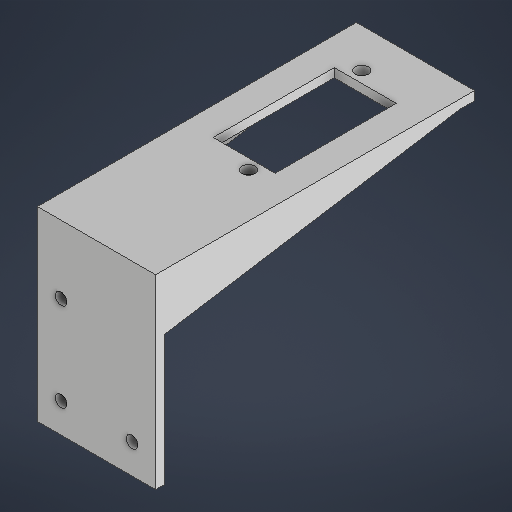
# Autodesk Inventor part: pan_base_holder_first_v1
Saved by Autodesk Inventor 2026 (Build 300175000, 175)
## iProperties
Created: 2025-06-27
Part Number: pan_base_holder_first_v1
Material: Generic
Document SubType Name: Modeling
Designer: user
Density: 1 g/cm^3
Appearance: Default
Author: user
Autodesk Inventor part; units mm, degrees
ref_plane "YZ Plane" through (0, 0, 0) normal (1, 0, 0) x (0, 1, 0)
ref_plane "XZ Plane" through (0, 0, 0) normal (0, 1, 0) x (-1, 0, 0)
ref_plane "XY Plane" through (0, 0, 0) normal (0, 0, 1) x (1, 0, 0)
sketch "Sketch1" plane through (0, 0, 0) normal (0, 0, 1) x (1, 0, 0)
  line L0 (-31, -31) -> (31, -31)
  line L1 (31, -31) -> (31, 31)
  line L2 (31, 31) -> (-31, 31)
  line L3 (-31, 31) -> (-31, -31)
  line L4 (-31, -31) -> (31, 31) construction
  line L5 (31, -31) -> (-31, 31) construction
  line L6 (-33, 33) -> (33, 33)
  line L7 (33, 33) -> (33, -33)
  line L8 (33, -33) -> (-33, -33)
  line L9 (-33, -33) -> (-33, 33)
  point P0 (0, 0)
  dimension "d0" = 62
  dimension "d1" = 62
  dimension "d2" = 2
  constraints: 20 end point, 4 parallel, 2 midpoint, 2 perpendicular, 1 horizontal, 3 other
  measures "d0" distance of L1.end L2.end
  measures "d1" distance of L0.end L1.end
  measures "d2" distance between parallel lines of L2 L6
extrude "Extrusion1" add sketch "Sketch1" along normal blind 2 contours L3 L2 L1 L0 | L6 L7 L8 L9
extrude "Extrusion2" add sketch "Sketch1" against normal blind 12
sketch "Sketch2" plane through (-33, 33, 2) normal (0, 1, 0) x (1, 0, 0)
  line L0 (13, 3) -> (53, 3)
  line L1 (53, 3) -> (53, 0)
  line L2 (53, 0) -> (13, 0)
  line L3 (13, 0) -> (13, 3)
  line L4 (0, 14) -> (0, 0) projected
  line L5 (0, 14) -> (66, 14) projected
  point P0 (33, 2)
  dimension "d7" = 40
  dimension "d8" = 3
  dimension "d9" = 13
  dimension "d10" = 11
  constraints: 8 end point, 2 parallel, 1 horizontal, 1 perpendicular
  measures "d7" distance of L1.end L2.end
  measures "d8" distance of L0.end L1.end
  measures "d9" distance between parallel lines of L4 L3
  measures "d10" distance between parallel lines of L5 L0
extrude "Extrusion3" add sketch "Sketch2" along normal blind 12
sketch "Sketch3" plane through (20, 33, -1) normal (0, 0, -1) x (-1, 0, 0)
  line L0 (40, 12) -> (0, 12) projected
  line L1 (40, 0) -> (40, 12) projected
  line L2 (0, 12) -> (40, 12)
  line L3 (40, 12) -> (40, 9)
  line L4 (40, 9) -> (0, 9)
  line L5 (0, 9) -> (0, 12)
  point P0 (20, -33)
  dimension "d13" = 3
  constraints: 8 end point, 2 parallel, 1 horizontal, 1 perpendicular, 1 point on line
  measures "d13" distance of L2.end L3.end
extrude "Extrusion4" add sketch "Sketch3" along normal blind 80
sketch "Sketch4" plane through (-20, 42, -1) normal (0, -1, 0) x (1, 0, 0)
  line L0 (30.5, -63) -> (9.5, -63)
  line L1 (9.5, -63) -> (9.5, -22)
  line L2 (9.5, -22) -> (30.5, -22)
  line L3 (30.5, -22) -> (30.5, -63)
  line L4 (40, 3) -> (40, -80) projected
  line L5 (0, 3) -> (40, 3) projected
  point P0 (20, 1)
  dimension "d16" = 21
  dimension "d17" = 41
  dimension "d18" = 9.5
  dimension "d19" = 25
  constraints: 8 end point, 2 parallel, 1 horizontal, 1 perpendicular
  measures "d16" distance of L0.start L0.end
  measures "d17" distance of L0.end L1.end
  measures "d18" distance between parallel lines of L4 L3
  measures "d19" distance between parallel lines of L2 L5
extrude "Extrusion5" cut sketch "Sketch4" against normal blind 80
sketch "Sketch5" plane through (-20, 42, -1) normal (0, -1, 0) x (1, 0, 0)
  line L0 (30.5, -63) -> (9.5, -63) projected
  line L1 (30.5, -63) -> (9.5, -63)
  line L2 (9.5, -63) -> (9.5, -70)
  line L3 (9.5, -70) -> (30.5, -70)
  line L4 (30.5, -70) -> (30.5, -63)
  circle A0 centre (15, -66.75) radius 2.25
  line L5 (30.5, -22) -> (30.5, -63) projected
  line L6 (30.5, -22) -> (9.5, -22)
  line L7 (9.5, -22) -> (9.5, -15)
  line L8 (9.5, -15) -> (30.5, -15)
  line L9 (30.5, -15) -> (30.5, -22)
  circle A1 centre (25, -18.5) radius 2.25
  point P0 (20, 1)
  point P1 (14.9217, -69.81)
  point P2 (13.9783, -69.81)
  point P3 (25.0283, -15.19)
  point P4 (25.9717, -15.19)
  dimension "d22" = 7
  dimension "d23" = 4.5
  dimension "d24" = 3.75
  dimension "d25" = 5.5
  dimension "d26" = 7
  dimension "d27" = 4.5
  dimension "d28" = 5.5
  dimension "d29" = 3.5
  constraints: 16 end point, 4 parallel, 2 centre point, 2 horizontal, 2 perpendicular
  measures "d22" distance of L2.end L1.end
  measures "d23" diameter of A0
  measures "d24" distance from line of A0.centre L0
  measures "d25" distance from line of L2 A0.centre
  measures "d26" distance of L6.end L7.end
  measures "d27" diameter of A1
  measures "d28" distance from line of L9 A1.centre
  measures "d29" distance from line of L6 A1.centre
extrude "Extrusion6" cut sketch "Sketch5" against normal blind 80 contours A0 | A1
sketch "Sketch6" plane through (-33, -33, 2) normal (0, -1, 0) x (1, 0, 0)
  line L0 (0, -14) -> (0, 0) projected
  line L1 (66, -14) -> (66, 0) projected
  line L2 (0, 0) -> (66, 0)
  line L3 (66, 0) -> (66, -14)
  line L4 (66, -14) -> (0, -14)
  line L5 (0, -14) -> (0, 0)
  point P0 (33, -2)
  point P1 (66, 0)
  constraints: 8 end point, 2 parallel, 1 horizontal, 1 perpendicular
extrude "Extrusion7" cut sketch "Sketch6" against normal up to surface (75 mm away)
sketch "Sketch7" plane through (0, 0, 2) normal (0, 0, 1) x (1, 0, 0)
  line L0 (-20, 42) -> (-20, 45) projected
  line L1 (20, 42) -> (20, 45) projected
  line L2 (-20, 45) -> (20, 45)
  line L3 (20, 45) -> (20, 42)
  line L4 (20, 42) -> (-20, 42)
  line L5 (-20, 42) -> (-20, 45)
  point P0 (0, 0)
  constraints: 8 end point, 2 parallel, 1 horizontal, 1 perpendicular
extrude "Extrusion8" add sketch "Sketch7" along normal blind 25
sketch "Sketch8" plane through (-20, 42, -81) normal (0, -1, 0) x (1, 0, 0)
  line L0 (0, 108) -> (0, 0) projected
  line L1 (40, 0) -> (40, 108) projected
  line L2 (0, 108) -> (40, 108)
  line L3 (40, 108) -> (40, 105)
  line L4 (40, 105) -> (0, 105)
  line L5 (0, 105) -> (0, 108)
  point P0 (20, 81)
  dimension "d36" = 3
  constraints: 8 end point, 2 parallel, 1 horizontal, 1 perpendicular, 1 point on line
  measures "d36" distance of L2.end L3.end
extrude "Extrusion9" add sketch "Sketch8" along normal blind 100
sketch "Sketch9" plane through (20, 42, 24) normal (0, 0, -1) x (-1, 0, 0)
  circle A0 centre (20, -90) radius 2
  circle A1 centre (8, -50) radius 2
  circle A2 centre (32, -20) radius 2
  line L0 (40, 0) -> (40, -100) projected
  line L1 (0, 0) -> (0, -100) projected
  line L2 (40, -100) -> (0, -100) projected
  line L3 (0, 0) -> (40, 0) projected
  point P0 (20, -42)
  dimension "d39" = 4
  dimension "d40" = 4
  dimension "d41" = 4
  dimension "d42" = 8
  dimension "d43" = 8
  dimension "d44" = 20
  dimension "d45" = 10
  dimension "d46" = 50
  dimension "d47" = 20
  constraints: 3 centre point
  measures "d39" diameter of A0
  measures "d40" diameter of A1
  measures "d41" diameter of A2
  measures "d42" distance from line of L0 A2.centre
  measures "d43" distance from line of L1 A1.centre
  measures "d44" distance from line of L0 A0.centre
  measures "d45" distance from line of L2 A0.centre
  measures "d46" distance from line of L2 A1.centre
  measures "d47" distance from line of L3 A2.centre
extrude "Extrusion10" cut sketch "Sketch9" against normal blind 10 contours A0 | A1 | A2
ref_plane "Work Plane1" through (0, 45, 27) normal (1, 0, 0) x (0, 0, -1)
sketch "Sketch11" plane through (20, 45, 27) normal (1, 0, 0) x (0, 0, -1)
  line L0 (3, -3) -> (3, -103) projected
  line L1 (3, -3) -> (103, -3)
  line L2 (103, -3) -> (103, -19)
  line L3 (103, -19) -> (3, -19)
  line L4 (3, -19) -> (3, -3)
  line L5 (103, -3) -> (3, -19)
  point P0 (27, -45)
  point P1 (3, -19)
  dimension "d55" = 100
  dimension "d56" = 16
  constraints: 10 end point, 2 parallel, 1 horizontal, 1 perpendicular
  measures "d55" distance of L2.end L3.end
  measures "d56" distance of L1.end L2.end
extrude "Extrusion12" add sketch "Sketch11" against normal blind 4 contours L1 L5 L0
ref_plane "Work Plane2" through (0, 45, -81) normal (-1, 0, 0) x (0, 0, 1)
mirror "Mirror1" about plane through (0, 45, -81) normal (-1, 0, 0) of "Extrusion12"
sketch "Sketch12" plane through (-20, -58, -81) normal (0, -1, 0) x (1, 0, 0)
  line L0 (0, 108) -> (0, 0) projected
  line L1 (40, 0) -> (40, 108) projected
  line L2 (0, 108) -> (40, 108)
  line L3 (40, 108) -> (40, 105)
  line L4 (40, 105) -> (0, 105)
  line L5 (0, 105) -> (0, 108)
  point P0 (20, 81)
  dimension "d59" = 3
  constraints: 8 end point, 2 parallel, 1 horizontal, 1 perpendicular, 1 point on line
  measures "d59" distance of L2.end L3.end
extrude "Extrusion13" cut sketch "Sketch12" against normal blind 40
sketch "Sketch13" plane through (20, 26, 24) normal (0, 0, -1) x (-1, 0, 0)
  circle A0 centre (32, -34) radius 2
  line L0 (0, -44) -> (40, -44) projected
  line L1 (40, 0) -> (40, -44) projected
  point P0 (20, -26)
  dimension "d62" = 4
  dimension "d63" = 10
  dimension "d64" = 8
  constraints: 1 centre point
  measures "d62" diameter of A0
  measures "d63" distance from line of L0 A0.centre
  measures "d64" distance from line of L1 A0.centre
extrude "Extrusion14" cut sketch "Sketch13" against normal blind 40
body "Solid1"
